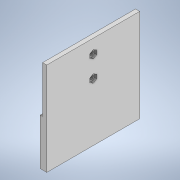
# Autodesk Inventor part: wallMountBottom
Saved by Autodesk Inventor 2021 (Build 250183000, 183)
## iProperties
Created: 2021-02-26
Part Number: wallMountBottom
Material: Generic
Document SubType Name: Modeling
Designer: jjaken
Density: 1 g/cm^3
Appearance: Default
Author: jjaken
Autodesk Inventor part; units mm, degrees
ref_plane "YZ Plane" through (0, 0, 0) normal (1, 0, 0) x (0, 1, 0)
ref_plane "XZ Plane" through (0, 0, 0) normal (0, 1, 0) x (-1, 0, 0)
ref_plane "XY Plane" through (0, 0, 0) normal (0, 0, 1) x (1, 0, 0)
sketch "Sketch1" plane through (0, 0, 0) normal (1, 0, 0) x (0, 1, 0)
  line L0 (50, 50) -> (-50, 50)
  line L1 (-50, 50) -> (-50, -50)
  line L2 (-50, -50) -> (50, -50)
  line L3 (50, -50) -> (50, 50)
  point P0 (0, 0)
  point P1 (50, 0)
  point P2 (0, -50)
  dimension "d0" = 100
  dimension "d1" = 100
  constraints: 8 end point, 2 midpoint, 2 parallel, 1 horizontal, 1 horizontal alignment, 1 perpendicular, 1 vertical alignment
  measures "d0" distance of L2.end L0.start
  measures "d1" distance of L1.end L2.end
extrude "Extrusion1" add sketch "Sketch1" along normal blind 4.5
sketch "Sketch2" plane through (0, 0, 0) normal (-1, 0, 0) x (0, 0, 1)
  line L0 (50, -50) -> (-50, -50) projected
  line L1 (50, 50) -> (50, -50) projected
  line L2 (-50, -50) -> (50, -50)
  line L3 (50, -50) -> (50, 0)
  line L4 (50, 0) -> (-50, 0)
  line L5 (-50, 0) -> (-50, -50)
  point P0 (0, 0)
  constraints: 8 end point, 2 parallel, 1 horizontal, 1 midpoint, 1 perpendicular
extrude "Extrusion2" add sketch "Sketch2" along normal blind 2.5
sketch "Sketch3" plane through (4.5, 0, 0) normal (1, 0, 0) x (0, 0, -1)
  line L0 (-50, -50) -> (50, -50) projected
  line L1 (50, -50) -> (50, 50) projected
  line L2 (50, 50) -> (-50, 50) projected
  line L3 (-50, 50) -> (-50, -50) projected
  point P0 (0, 0)
  point P1 (0, 35)
  point P2 (0, 12.5)
  point P3 (0, 50)
  dimension "d6" = 37.5
  dimension "d7" = 15
  constraints: 2 vertical alignment, 1 midpoint
  measures "d6" distance from line of point (0, 12.5) L2
  measures "d7" distance from line of point (0, 35) L2
hole "Hole1" at (4.5, 35, 0) at (4.5, 12.5, 0) direction (-1, 0, 0) diameter 4.5 end through all
sketch "Sketch4" plane through (4.5, 0, 0) normal (1, 0, 0) x (0, 0, -1)
  circle A0 centre (0, 35) radius 2.25 projected
  circle A1 centre (0, 12.5) radius 2.25 projected
  line L0 (-50, -50) -> (50, -50) projected
  line L1 (50, -50) -> (50, 50) projected
  line L2 (50, 50) -> (-50, 50) projected
  line L3 (-50, 50) -> (-50, -50) projected
  line L4 (3.75, 10.3349) -> (0, 8.1699)
  line L5 (0, 8.1699) -> (-3.75, 10.3349)
  line L6 (-3.75, 10.3349) -> (-3.75, 14.6651)
  line L7 (-3.75, 14.6651) -> (0, 16.8301)
  line L8 (0, 16.8301) -> (3.75, 14.6651)
  line L9 (3.75, 14.6651) -> (3.75, 10.3349)
  line L10 (3.75, 32.8349) -> (0, 30.6699)
  line L11 (0, 30.6699) -> (-3.75, 32.8349)
  line L12 (-3.75, 32.8349) -> (-3.75, 37.1651)
  line L13 (-3.75, 37.1651) -> (0, 39.3301)
  line L14 (0, 39.3301) -> (3.75, 37.1651)
  line L15 (3.75, 37.1651) -> (3.75, 32.8349)
  point P0 (0, 0)
  dimension "d15" = 7.5
  dimension "d16" = 7.5
  constraints: 24 end point, 2 coincident, 2 parallel, 26 other
  measures "d15" distance between parallel lines of L15 L12
  measures "d16" distance between parallel lines of L6 L9
extrude "Extrusion3" cut sketch "Sketch4" against normal blind 2.25 contours L4 L5 L6 L7 L8 L9 | L10 L11 L12 L13 L14 L15
equation "\"d16\" = d15"
body "Solid1"
